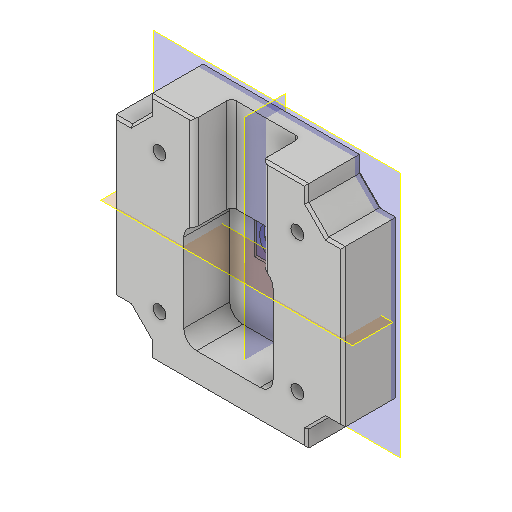
# Autodesk Inventor part: 20_Cube_Insert_SEEED_Xiao_Sense_Camera
Saved by Autodesk Inventor 2022 (Build 260153000, 153)
## iProperties
Created: 2019-07-01
Part Number: 20_Cube_Insert_SEEED_Xiao_Sense_Camera
Material: Generic
Document SubType Name: Modeling
Designer: diederichbenedict
Density: 1 g/cm^3
Appearance: Default
Author: diederichbenedict
Autodesk Inventor part; units mm, degrees
ref_plane "YZ Plane" through (0, 0, 0) normal (1, 0, 0) x (0, 1, 0)
ref_plane "Work Plane1" through (-56.3599, 0, 22) normal (0, 0, -1) x (-1, 0, 0)
sketch "Sketch1" plane through (-56.3599, 0, 22) normal (0, 0, -1) x (-1, 0, 0)
  line L0 (-4.0299, -0.3538) -> (-2.2322, 1.4439) construction
  arc A0 (-1.4439, 2.2322) -> (-2.2322, 1.4439) centre (-0.9299, 0.9299) ccw construction
  line L1 (-1.4439, 2.2322) -> (0.3538, 4.0299) construction
  line L2 (-37.8299, 42.8299) -> (-37.8299, 37.8299) construction
  line L3 (-37.8299, 37.8299) -> (-42.9208, 37.8299) construction
  line L4 (-37.8299, 42.2137) -> (-37.8299, 45.8299) construction
  line L5 (-37.8299, 45.8299) -> (-4.0299, 45.8299) construction
  line L6 (-4.0299, 45.8299) -> (-4.0299, 42.2137) construction
  line L7 (-4.0299, 4.0299) -> (0.3538, 4.0299) projected
  circle A1 centre (-20.9299, 20.9299) radius 17.5 projected
  line L8 (-20.9299, 58.9723) -> (17.1124, 20.9299) construction
  line L9 (17.1124, 20.9299) -> (-20.9299, -17.1124) construction
  line L10 (-20.9299, -17.1124) -> (-58.9723, 20.9299) construction
  line L11 (-58.9723, 20.9299) -> (-20.9299, 58.9723) construction
  line L12 (-20.9299, 58.9723) -> (-20.9299, -17.1124) construction
  line L13 (17.1124, 20.9299) -> (-58.9723, 20.9299) construction
  line L14 (-20.9299, 58.9723) -> (32.8701, 58.9723) construction
  line L15 (-43.4299, 43.4299) -> (1.5701, 43.4299) construction
  line L16 (1.5701, 43.4299) -> (1.5701, -1.5701) construction
  line L17 (1.5701, -1.5701) -> (-43.4299, -1.5701) construction
  line L18 (-43.4299, -1.5701) -> (-43.4299, 43.4299) construction
  line L19 (-43.4299, 43.4299) -> (1.5701, -1.5701) construction
  line L20 (1.5701, 43.4299) -> (-43.4299, -1.5701) construction
  line L21 (-43.4299, 5.3876) -> (-43.4299, 36.4723)
  line L22 (-43.4299, 36.4723) -> (-36.4723, 43.4299)
  line L23 (-36.4723, 43.4299) -> (-5.3876, 43.4299)
  line L24 (-5.3876, 43.4299) -> (1.5701, 36.4723)
  line L25 (1.5701, 36.4723) -> (1.5701, 5.3876)
  line L26 (1.5701, 5.3876) -> (-5.3876, -1.5701)
  line L27 (-5.3876, -1.5701) -> (-36.4723, -1.5701)
  line L28 (-36.4723, -1.5701) -> (-43.4299, 5.3876)
  line L29 (-4.0299, 42.2137) -> (-37.8299, 42.2137) projected
  line L30 (-4.0299, -0.3538) -> (-4.0299, 4.0299) projected
  circle A2 centre (-20.9299, 20.9299) radius 1.5
  line L31 (-10.9299, 10.9299) -> (-30.9299, 10.9299) construction
  line L32 (-30.9299, 10.9299) -> (-30.9299, 30.9299) construction
  line L33 (-30.9299, 30.9299) -> (-10.9299, 30.9299) construction
  line L34 (-10.9299, 30.9299) -> (-10.9299, 10.9299) construction
  line L35 (-10.9299, 10.9299) -> (-30.9299, 30.9299) construction
  line L36 (-30.9299, 10.9299) -> (-10.9299, 30.9299) construction
  circle A3 centre (-30.9299, 30.9299) radius 1.4
  circle A4 centre (-30.9299, 10.9299) radius 1.4
  circle A5 centre (-10.9299, 10.9299) radius 1.4
  line L37 (-45.8299, 37.8299) -> (-42.0723, 37.8299) construction
  line L38 (-42.1723, 37.7299) -> (-45.8299, 37.7299)
  line L39 (-45.8299, 37.7299) -> (-45.8299, 4.1299)
  line L40 (-45.8299, 4.1299) -> (-42.1723, 4.1299)
  line L41 (-42.1723, 4.1299) -> (-42.1723, 37.7299)
  line L42 (-45.8299, 4.0299) -> (-42.0723, 4.0299) construction
  line L43 (-45.8299, 37.8299) -> (-42.0723, 37.8299) projected
  line L44 (-37.7299, 45.8299) -> (-4.1299, 45.8299)
  line L45 (-4.1299, 45.8299) -> (-4.1299, 42.1723)
  line L46 (-4.1299, 42.1723) -> (-37.7299, 42.1723)
  line L47 (-37.7299, 42.1723) -> (-37.7299, 45.8299)
  line L48 (0.4701, 37.8299) -> (0.4701, 4.0299) construction
  line L49 (0.4701, 4.0299) -> (3.9701, 4.0299) construction
  line L50 (3.9701, 37.8299) -> (3.9701, 4.0299) construction
  line L51 (0.4701, 37.8299) -> (3.9701, 37.8299) construction
  line L52 (-45.8299, -3.9701) -> (-4.0299, -3.9701) construction
  line L53 (0.3124, 37.7299) -> (3.9701, 37.7299)
  line L54 (3.9701, 37.7299) -> (3.9701, 4.1299)
  line L55 (3.9701, 4.1299) -> (0.3124, 4.1299)
  line L56 (0.3124, 4.1299) -> (0.3124, 37.7299)
  line L57 (-4.1713, -0.3538) -> (-37.7299, -0.3538)
  line L58 (-37.7299, -0.3538) -> (-37.7299, -3.9701)
  line L59 (-37.7299, -3.9701) -> (-4.1713, -3.9701)
  line L60 (-4.1713, -3.9701) -> (-4.1713, -0.3538)
  point P0 (-37.8299, 4.0299)
  dimension "d18" = 53.8
  dimension "d19" = 45
  dimension "d20" = 53.8
  dimension "d21" = 45
  dimension "d22" = 45
  dimension "d30" = 20
  dimension "d31" = 20
  dimension "d32" = 2.8
  dimension "d33" = 2.8
  dimension "d34" = 2.8
  dimension "d35" = 3
  dimension "d36" = 0.1
  dimension "d37" = 0.1
  dimension "d38" = 0.1
  dimension "d39" = 0.1
  constraints: 86 end point, 21 point on line, 14 parallel, 8 perpendicular, 7 horizontal, 7 midpoint, 4 centre point, 4 coincident, 1 equal length
  measures "d18" distance of L8.start L8.end
  measures "d19" angle of L8 L14
  measures "d20" distance of L8.end L9.end
  measures "d21" distance of L16.end L17.end
  measures "d22" distance of L15.end L16.end
  measures "d30" distance of L32.end L33.end
  measures "d31" distance of L31.end L32.end
  measures "d32" diameter of A3
  measures "d33" diameter of A4
  measures "d34" diameter of A5
  measures "d35" diameter of A2
  measures "d36" distance between parallel lines of L38 L43
  measures "d37" distance between parallel lines of L40 L42
  measures "d38" distance between parallel lines of L45 L6
  measures "d39" distance between parallel lines of L4 L47
extrude "Extrusion1" add sketch "Sketch1" along normal blind 12 contours L30 L26 L57 L28 L41 L22 L46 L24 L56 L7 | L7 L26 L30 | L56 L24 L25 L26 | L26 L25 L24 L53 L54 L55 | L60 L59 L58 L57 L28 L27 L26 | L26 L27 L28 L57 | L46 L22 L29 L24 | L24 L29 L45 | L40 L39 L38 L22 L21 L28 | L28 L21 L22 L41 | L29 L22 L23 L24 | L24 L23 L22 L29 L47 L44 L45 | L47 L29 L22 | A1 | A2 | A3 | A4 | A5
sketch "Skizze4" plane through (-56.3599, 0, 10) normal (0, 0, -1) x (-1, 0, 0)
  line L0 (-37.7299, 42.1723) -> (-42.1723, 37.7299) projected
  line L1 (-42.1723, 37.7299) -> (-45.8299, 37.7299) projected
  line L2 (-45.8299, 37.7299) -> (-45.8299, 4.1299) construction
  line L3 (-45.8299, 4.1299) -> (-42.1723, 4.1299) projected
  line L4 (-42.1723, 4.1299) -> (-37.6885, -0.3538) projected
  line L5 (-37.6885, -0.3538) -> (-37.7299, -0.3538) projected
  line L6 (-37.7299, -0.3538) -> (-37.7299, -3.9701) projected
  line L7 (-37.7299, -3.9701) -> (-4.1713, -3.9701) construction
  line L8 (-4.1713, -3.9701) -> (-4.1713, -0.3538) projected
  line L9 (-4.1713, -0.3538) -> (0.3124, 4.1299) projected
  line L10 (0.3124, 4.1299) -> (3.9701, 4.1299) projected
  line L11 (3.9701, 4.1299) -> (3.9701, 37.7299) construction
  line L12 (3.9701, 37.7299) -> (0.3124, 37.7299) projected
  line L13 (0.3124, 37.7299) -> (-4.1299, 42.1723) projected
  line L14 (-4.1299, 42.1723) -> (-4.1299, 45.8299) projected
  line L15 (-4.1299, 45.8299) -> (-37.7299, 45.8299) construction
  line L16 (-37.7299, 45.8299) -> (-37.7299, 42.1723) projected
  line L17 (-37.9299, 46.0299) -> (-3.9299, 46.0299) construction
  line L18 (-3.9299, 46.0299) -> (-3.9299, 42.2551)
  line L19 (-3.9299, 42.2551) -> (0.3953, 37.9299)
  line L20 (0.3953, 37.9299) -> (4.1701, 37.9299)
  line L21 (4.1701, 37.9299) -> (4.1701, 3.9299) construction
  line L22 (4.1701, 3.9299) -> (0.3953, 3.9299)
  line L23 (0.3953, 3.9299) -> (-3.9713, -0.4367)
  line L24 (-3.9713, -0.4367) -> (-3.9713, -4.1701)
  line L25 (-3.9713, -4.1701) -> (-37.9299, -4.1701) construction
  line L26 (-37.9299, -4.1701) -> (-37.9299, -0.3953)
  line L27 (-37.9299, -0.3953) -> (-42.2551, 3.9299)
  line L28 (-42.2551, 3.9299) -> (-46.0299, 3.9299)
  line L29 (-46.0299, 3.9299) -> (-46.0299, 37.9299) construction
  line L30 (-46.0299, 37.9299) -> (-42.2551, 37.9299)
  line L31 (-42.2551, 37.9299) -> (-37.9299, 42.2551)
  line L32 (-37.9299, 42.2551) -> (-37.9299, 46.0299)
  line L33 (-45.8299, 37.7299) -> (-45.8299, 37.9299)
  line L34 (-4.1299, 45.8299) -> (-37.7299, 45.8299) projected
  line L35 (-37.7299, 45.8299) -> (-37.9299, 45.8299)
  line L36 (-4.1299, 45.8299) -> (-3.9299, 45.8299)
  line L37 (3.9701, 37.7299) -> (3.9701, 37.9299)
  line L38 (3.9701, 4.1299) -> (3.9701, 37.7299) projected
  line L39 (3.9701, 4.1299) -> (3.9701, 3.9299)
  line L40 (-4.1713, -3.9701) -> (-3.9713, -3.9701)
  line L41 (-37.7299, -3.9701) -> (-37.9299, -3.9701)
  line L42 (-45.8299, 4.1299) -> (-45.8299, 3.9299)
  point P0 (-56.3599, 0)
  dimension "d40" = 0.2
  constraints: 48 end point, 12 point on line, 4 perpendicular, 15 other
  measures "d40" distance between parallel lines of L15 L17
extrude "IM_offset" add sketch "Skizze4" against normal up to surface (12 mm away)
ref_plane "Arbeitsebene5" through (-35.4299, 3.9299, 22) normal (-1, 0, 0) x (0, 0, 1)
ref_plane "Arbeitsebene6" through (-18.4299, 20.9299, 22) normal (0, 1, 0) x (-1, 0, 0)
sketch "Skizze31" plane through (-56.3599, 0, 10) normal (0, 0, -1) x (-1, 0, 0)
  line L0 (3.9701, 3.9299) -> (3.9701, 37.9299) projected
  line L1 (3.9701, 37.9299) -> (0.3953, 37.9299) projected
  line L2 (0.3953, 37.9299) -> (-3.9299, 42.2551) projected
  line L3 (-3.9299, 42.2551) -> (-3.9299, 45.8299) projected
  line L4 (-3.9299, 45.8299) -> (-37.9299, 45.8299) projected
  line L5 (-37.9299, 45.8299) -> (-37.9299, 42.2551) projected
  line L6 (-37.9299, 42.2551) -> (-42.2551, 37.9299) projected
  line L7 (-42.2551, 37.9299) -> (-45.8299, 37.9299) projected
  line L8 (-45.8299, 37.9299) -> (-45.8299, 3.9299) projected
  line L9 (-42.2551, 3.9299) -> (-45.8299, 3.9299) projected
  line L10 (-37.9299, -0.3953) -> (-42.2551, 3.9299) projected
  line L11 (-37.9299, -3.9701) -> (-37.9299, -0.3953) projected
  line L12 (-3.9713, -3.9701) -> (-37.9299, -3.9701) projected
  line L13 (-3.9713, -3.9701) -> (-3.9713, -0.4367) projected
  line L14 (-3.9713, -0.4367) -> (0.3953, 3.9299) projected
  line L15 (0.3953, 3.9299) -> (3.9701, 3.9299) projected
  circle A0 centre (-20.9506, 20.9092) radius 3.75
  point P0 (-56.3599, 0)
  dimension "d181" = 7.5
  constraints: 1 centre point
  measures "d181" diameter of A0
extrude "Extrusion26" cut sketch "Skizze31" against normal blind 10 contours A0
chamfer "Fase2" distance 0.5 angle 45 33 edges at (-35.4299, 45.8299, 22) (-18.4299, 44.0425, 22) (-16.2673, 40.0925, 22) (-12.3173, 37.9299, 22) (-10.5299, 20.9299, 22) (-12.3173, 3.9299, 22) (-16.2673, 1.7673, 22) (-18.4299, -2.1827, 22) (-35.4092, -3.9701, 22) (-52.3885, -2.2034, 22) (-54.5718, 1.7466, 22) (-58.5425, 3.9299, 22) (-60.3299, 20.9299, 22) (-58.5425, 37.9299, 22) (-54.5925, 40.0925, 22) (-54.5718, 1.7466, 10) (-58.5425, 3.9299, 10) (-60.3299, 20.9299, 10) (-52.3885, -2.2034, 10) (-35.4092, -3.9701, 10) (-18.4299, -2.1827, 10) (-16.2673, 1.7673, 10) (-12.3173, 3.9299, 10) (-10.5299, 20.9299, 10) (-12.3173, 37.9299, 10) (-16.2673, 40.0925, 10) (-18.4299, 44.0425, 10) (-35.4299, 45.8299, 10) (-52.4299, 44.0425, 10) (-54.5925, 40.0925, 10) (-58.5425, 37.9299, 10) (-31.6592, 20.9092, 10) (-52.4299, 44.0425, 22)
ref_plane "Arbeitsebene9" through (-56.3599, 0, 11.5) normal (0, 0, -1) x (-1, 0, 0)
sketch "Skizze34" plane through (-56.3599, 0, 11.5) normal (0, 0, -1) x (-1, 0, 0)
  circle A0 centre (-20.9299, 20.9299) radius 4 projected
  line L0 (-16.6299, 25.2299) -> (-25.2299, 25.2299)
  line L1 (-25.2299, 25.2299) -> (-25.2299, 16.6299)
  line L2 (-25.2299, 16.6299) -> (-16.6299, 16.6299)
  line L3 (-16.6299, 16.6299) -> (-16.6299, 25.2299)
  line L4 (-16.6299, 25.2299) -> (-25.2299, 16.6299) construction
  line L5 (-25.2299, 25.2299) -> (-16.6299, 16.6299) construction
  point P0 (-56.3599, 0)
  dimension "d194" = 8.6
  dimension "d195" = 8.6
  constraints: 12 end point, 2 midpoint, 2 parallel, 1 horizontal, 1 perpendicular
  measures "d194" distance of L2.end L1.end
  measures "d195" distance of L1.end L0.end
extrude "Extrusion29" cut sketch "Skizze34" against normal through all contours A0 | L3 L2 L1 L0
sketch "Skizze35" plane through (-56.3599, 0, 22) normal (0, 0, 1) x (1, 0, 0)
  arc A0 (29.8299, 22.6299) -> (27.8299, 24.6299) centre (27.8299, 22.6299) ccw projected
  line L0 (27.8299, 24.6299) -> (14.0299, 24.6299) projected
  arc A1 (14.0299, 24.6299) -> (12.0299, 22.6299) centre (14.0299, 22.6299) ccw projected
  line L1 (12.0299, 22.6299) -> (12.0299, 22.5499) projected
  line L2 (12.0299, 22.5499) -> (13.3099, 22.5499) projected
  arc A2 (13.3099, 20.7499) -> (13.3099, 22.5499) centre (13.3099, 21.6499) ccw projected
  line L3 (13.3099, 20.7499) -> (12.0299, 20.7499) projected
  line L4 (12.0299, 20.7499) -> (12.0299, 20.0099) projected
  line L5 (12.0299, 20.0099) -> (13.3099, 20.0099) projected
  arc A3 (13.3099, 18.2099) -> (13.3099, 20.0099) centre (13.3099, 19.1099) ccw projected
  line L6 (13.3099, 18.2099) -> (12.0299, 18.2099) projected
  line L7 (12.0299, 18.2099) -> (12.0299, 17.4699) projected
  line L8 (12.0299, 17.4699) -> (13.3099, 17.4699) projected
  arc A4 (13.3099, 15.6699) -> (13.3099, 17.4699) centre (13.3099, 16.5699) ccw projected
  line L9 (13.3099, 15.6699) -> (12.0299, 15.6699) projected
  line L10 (12.0299, 15.6699) -> (12.0299, 14.9299) projected
  line L11 (12.0299, 14.9299) -> (13.3099, 14.9299) projected
  arc A5 (13.3099, 13.1299) -> (13.3099, 14.9299) centre (13.3099, 14.0299) ccw projected
  line L12 (13.3099, 13.1299) -> (12.0299, 13.1299) projected
  line L13 (12.0299, 13.1299) -> (12.0299, 12.3899) projected
  line L14 (12.0299, 12.3899) -> (13.3099, 12.3899) projected
  arc A6 (13.3099, 10.5899) -> (13.3099, 12.3899) centre (13.3099, 11.4899) ccw projected
  line L15 (13.3099, 10.5899) -> (12.0299, 10.5899) projected
  line L16 (12.0299, 10.5899) -> (12.0299, 9.8499) projected
  line L17 (12.0299, 9.8499) -> (13.3099, 9.8499) projected
  arc A7 (13.3099, 8.0499) -> (13.3099, 9.8499) centre (13.3099, 8.9499) ccw projected
  line L18 (13.3099, 8.0499) -> (12.0299, 8.0499) projected
  line L19 (12.0299, 8.0499) -> (12.0299, 7.3099) projected
  line L20 (12.0299, 7.3099) -> (13.3099, 7.3099) projected
  arc A8 (13.3099, 5.5099) -> (13.3099, 7.3099) centre (13.3099, 6.4099) ccw projected
  line L21 (13.3099, 5.5099) -> (12.0299, 5.5099) projected
  line L22 (12.0299, 5.5099) -> (12.0299, 5.4299) projected
  arc A9 (12.0299, 5.4299) -> (14.0299, 3.4299) centre (14.0299, 5.4299) ccw projected
  line L23 (14.0299, 3.4299) -> (27.8299, 3.4299) projected
  arc A10 (27.8299, 3.4299) -> (29.8299, 5.4299) centre (27.8299, 5.4299) ccw projected
  line L24 (29.8299, 5.4299) -> (29.8299, 5.5099) projected
  line L25 (29.8299, 5.5099) -> (28.5499, 5.5099) projected
  arc A11 (28.5499, 7.3099) -> (28.5499, 5.5099) centre (28.5499, 6.4099) ccw projected
  line L26 (28.5499, 7.3099) -> (29.8299, 7.3099) projected
  line L27 (29.8299, 7.3099) -> (29.8299, 8.0499) projected
  line L28 (29.8299, 8.0499) -> (28.5499, 8.0499) projected
  arc A12 (28.5499, 9.8499) -> (28.5499, 8.0499) centre (28.5499, 8.9499) ccw projected
  line L29 (28.5499, 9.8499) -> (29.8299, 9.8499) projected
  line L30 (29.8299, 9.8499) -> (29.8299, 10.5899) projected
  line L31 (29.8299, 10.5899) -> (28.5499, 10.5899) projected
  arc A13 (28.5499, 12.3899) -> (28.5499, 10.5899) centre (28.5499, 11.4899) ccw projected
  line L32 (28.5499, 12.3899) -> (29.8299, 12.3899) projected
  line L33 (29.8299, 12.3899) -> (29.8299, 13.1299) projected
  line L34 (29.8299, 13.1299) -> (28.5499, 13.1299) projected
  arc A14 (28.5499, 14.9299) -> (28.5499, 13.1299) centre (28.5499, 14.0299) ccw projected
  line L35 (28.5499, 14.9299) -> (29.8299, 14.9299) projected
  line L36 (29.8299, 14.9299) -> (29.8299, 15.6699) projected
  line L37 (29.8299, 15.6699) -> (28.5499, 15.6699) projected
  arc A15 (28.5499, 17.4699) -> (28.5499, 15.6699) centre (28.5499, 16.5699) ccw projected
  line L38 (28.5499, 17.4699) -> (29.8299, 17.4699) projected
  line L39 (29.8299, 17.4699) -> (29.8299, 18.2099) projected
  line L40 (29.8299, 18.2099) -> (28.5499, 18.2099) projected
  arc A16 (28.5499, 20.0099) -> (28.5499, 18.2099) centre (28.5499, 19.1099) ccw projected
  line L41 (28.5499, 20.0099) -> (29.8299, 20.0099) projected
  line L42 (29.8299, 20.0099) -> (29.8299, 20.7499) projected
  line L43 (29.8299, 20.7499) -> (28.5499, 20.7499) projected
  arc A17 (28.5499, 22.5499) -> (28.5499, 20.7499) centre (28.5499, 21.6499) ccw projected
  line L44 (28.5499, 22.5499) -> (29.8299, 22.5499) projected
  line L45 (29.8299, 22.5499) -> (29.8299, 22.6299) projected
  line L46 (29.8299, 22.5499) -> (12.0299, 22.5499)
  line L47 (12.0299, 22.5499) -> (12.0299, 5.4299)
  line L48 (12.0299, 5.4299) -> (29.8299, 5.4299)
  line L49 (29.8299, 5.4299) -> (29.8299, 22.5499)
  line L50 (27.8299, 2.6225) -> (14.0299, 2.6225)
  arc A18 (11.2225, 5.4299) -> (14.0299, 2.6225) centre (14.0299, 5.4299) ccw
  line L51 (11.2225, 5.4299) -> (11.2225, 6.3173)
  line L52 (11.2225, 6.3173) -> (13.3099, 6.3173)
  arc A19 (13.3099, 6.3173) -> (13.3099, 6.5025) centre (13.3099, 6.4099) ccw
  line L53 (13.3099, 6.5025) -> (11.2225, 6.5025)
  line L54 (11.2225, 6.5025) -> (11.2225, 8.8573)
  line L55 (11.2225, 8.8573) -> (13.3099, 8.8573)
  arc A20 (13.3099, 8.8573) -> (13.3099, 9.0425) centre (13.3099, 8.9499) ccw
  line L56 (13.3099, 9.0425) -> (11.2225, 9.0425)
  line L57 (11.2225, 9.0425) -> (11.2225, 11.3973)
  line L58 (11.2225, 11.3973) -> (13.3099, 11.3973)
  arc A21 (13.3099, 11.3973) -> (13.3099, 11.5825) centre (13.3099, 11.4899) ccw
  line L59 (13.3099, 11.5825) -> (11.2225, 11.5825)
  line L60 (11.2225, 11.5825) -> (11.2225, 13.9373)
  line L61 (11.2225, 13.9373) -> (13.3099, 13.9373)
  arc A22 (13.3099, 13.9373) -> (13.3099, 14.1225) centre (13.3099, 14.0299) ccw
  line L62 (13.3099, 14.1225) -> (11.2225, 14.1225)
  line L63 (11.2225, 14.1225) -> (11.2225, 16.4773)
  line L64 (11.2225, 16.4773) -> (13.3099, 16.4773)
  arc A23 (13.3099, 16.4773) -> (13.3099, 16.6625) centre (13.3099, 16.5699) ccw
  line L65 (13.3099, 16.6625) -> (11.2225, 16.6625)
  line L66 (11.2225, 16.6625) -> (11.2225, 19.0173)
  line L67 (11.2225, 19.0173) -> (13.3099, 19.0173)
  arc A24 (13.3099, 19.0173) -> (13.3099, 19.2025) centre (13.3099, 19.1099) ccw
  line L68 (13.3099, 19.2025) -> (11.2225, 19.2025)
  line L69 (11.2225, 19.2025) -> (11.2225, 21.5573)
  line L70 (11.2225, 21.5573) -> (13.3099, 21.5573)
  arc A25 (13.3099, 21.5573) -> (13.3099, 21.7425) centre (13.3099, 21.6499) ccw
  line L71 (13.3099, 21.7425) -> (11.2225, 21.7425)
  line L72 (11.2225, 21.7425) -> (11.2225, 22.6299)
  arc A26 (14.0299, 25.4373) -> (11.2225, 22.6299) centre (14.0299, 22.6299) ccw
  line L73 (14.0299, 25.4373) -> (27.8299, 25.4373)
  arc A27 (30.6373, 22.6299) -> (27.8299, 25.4373) centre (27.8299, 22.6299) ccw
  line L74 (30.6373, 22.6299) -> (30.6373, 21.7425)
  line L75 (30.6373, 21.7425) -> (28.5499, 21.7425)
  arc A28 (28.5499, 21.7425) -> (28.5499, 21.5573) centre (28.5499, 21.6499) ccw
  line L76 (28.5499, 21.5573) -> (30.6373, 21.5573)
  line L77 (30.6373, 21.5573) -> (30.6373, 19.2025)
  line L78 (30.6373, 19.2025) -> (28.5499, 19.2025)
  arc A29 (28.5499, 19.2025) -> (28.5499, 19.0173) centre (28.5499, 19.1099) ccw
  line L79 (28.5499, 19.0173) -> (30.6373, 19.0173)
  line L80 (30.6373, 19.0173) -> (30.6373, 16.6625)
  line L81 (30.6373, 16.6625) -> (28.5499, 16.6625)
  arc A30 (28.5499, 16.6625) -> (28.5499, 16.4773) centre (28.5499, 16.5699) ccw
  line L82 (28.5499, 16.4773) -> (30.6373, 16.4773)
  line L83 (30.6373, 16.4773) -> (30.6373, 14.1225)
  line L84 (30.6373, 14.1225) -> (28.5499, 14.1225)
  arc A31 (28.5499, 14.1225) -> (28.5499, 13.9373) centre (28.5499, 14.0299) ccw
  line L85 (28.5499, 13.9373) -> (30.6373, 13.9373)
  line L86 (30.6373, 13.9373) -> (30.6373, 11.5825)
  line L87 (30.6373, 11.5825) -> (28.5499, 11.5825)
  arc A32 (28.5499, 11.5825) -> (28.5499, 11.3973) centre (28.5499, 11.4899) ccw
  line L88 (28.5499, 11.3973) -> (30.6373, 11.3973)
  line L89 (30.6373, 11.3973) -> (30.6373, 9.0425)
  line L90 (30.6373, 9.0425) -> (28.5499, 9.0425)
  arc A33 (28.5499, 9.0425) -> (28.5499, 8.8573) centre (28.5499, 8.9499) ccw
  line L91 (28.5499, 8.8573) -> (30.6373, 8.8573)
  line L92 (30.6373, 8.8573) -> (30.6373, 6.5025)
  line L93 (30.6373, 6.5025) -> (28.5499, 6.5025)
  arc A34 (28.5499, 6.5025) -> (28.5499, 6.3173) centre (28.5499, 6.4099) ccw
  line L94 (28.5499, 6.3173) -> (30.6373, 6.3173)
  line L95 (30.6373, 6.3173) -> (30.6373, 5.4299)
  arc A35 (27.8299, 2.6225) -> (30.6373, 5.4299) centre (27.8299, 5.4299) ccw
  line L96 (30.6373, 6.3173) -> (11.2225, 6.3173)
  line L97 (11.2225, 6.3173) -> (11.2225, 21.7425)
  line L98 (11.2225, 21.7425) -> (30.6373, 21.7425)
  line L99 (30.6373, 21.7425) -> (30.6373, 6.3173)
  point P0 (56.3599, 0)
  point P1 (11.2225, 21.5573)
  point P2 (11.2225, 19.2025)
  point P3 (11.2225, 19.0173)
  point P4 (11.2225, 16.6625)
  point P5 (11.2225, 16.4773)
  point P6 (11.2225, 14.1225)
  point P7 (11.2225, 13.9373)
  point P8 (11.2225, 11.5825)
  point P9 (11.2225, 11.3973)
  point P10 (11.2225, 9.0425)
  point P11 (11.2225, 8.8573)
  point P12 (11.2225, 6.5025)
  point P13 (11.2225, 6.3173)
  point P14 (30.6373, 6.5025)
  point P15 (30.6373, 19.2025)
  constraints: 108 end point, 36 point on circle, 18 centre point, 4 parallel, 2 horizontal, 2 perpendicular, 63 other
extrude "Extrusion30" cut sketch "Skizze35" against normal blind 10
sketch "Skizze36" plane through (-52.4299, 45.8299, 10.5) normal (0, 1, 0) x (1, 0, 0)
  arc A0 (20.5, -9.5) -> (21.5, -8.5) centre (20.5, -8.5) ccw projected
  arc A1 (12.5, -8.5) -> (13.5, -9.5) centre (13.5, -8.5) ccw projected
  arc A2 (21.5, -7.33) -> (20.5, -6.33) centre (20.5, -7.33) ccw projected
  arc A3 (13.5, -6.33) -> (12.5, -7.33) centre (13.5, -7.33) ccw projected
  line L0 (20.5, -8.5) -> (13.5, -8.5)
  line L1 (13.5, -8.5) -> (13.5, -7.33)
  line L2 (13.5, -7.33) -> (20.5, -7.33)
  line L3 (20.5, -7.33) -> (20.5, -8.5)
  line L4 (9.5, -12.5) -> (24.5, -12.5)
  line L5 (24.5, -12.5) -> (24.5, -3.33)
  line L6 (24.5, -3.33) -> (9.5, -3.33)
  line L7 (9.5, -3.33) -> (9.5, -12.5)
  point P0 (52.4299, 10.5)
  dimension "d200" = 4
  constraints: 16 end point, 4 parallel, 2 perpendicular, 1 horizontal, 3 other
  measures "d200" distance between parallel lines of L0 L4
ref_plane "Arbeitsebene10" through (-41.4299, 4.7299, 19.7) normal (0, -1, 0) x (1, 0, 0)
extrude "Extrusion31" cut sketch "Skizze36" against normal up to surface (41.1 mm away) contours L0 L1 L2 L3 | L7 L6 L5 L4
fillet "Rundung3" radius 1 4 edges at (-27.9299, 35.3512, 22) (-27.9299, 35.6012, 13.83) (-42.9299, 35.3512, 22) (-42.9299, 35.6012, 13.83)
sketch "Skizze37" plane through (-56.3599, 0, 22) normal (0, 0, 1) x (1, 0, 0)
  line L0 (12.4299, 45.3299) -> (12.4299, 24.9368) projected
  line L1 (4.4299, 45.3299) -> (12.4299, 45.3299) projected
  line L2 (4.4299, 42.048) -> (4.4299, 45.3299) projected
  line L3 (-0.1882, 37.4299) -> (4.4299, 42.048) projected
  line L4 (-3.4701, 37.4299) -> (-0.1882, 37.4299) projected
  line L5 (-3.4701, 4.4299) -> (-3.4701, 37.4299) projected
  line L6 (-0.1882, 4.4299) -> (-3.4701, 4.4299) projected
  line L7 (4.4713, -0.2296) -> (-0.1882, 4.4299) projected
  line L8 (4.4713, -3.4701) -> (4.4713, -0.2296) projected
  line L9 (37.4299, -3.4701) -> (4.4713, -3.4701) projected
  line L10 (37.4299, -0.1882) -> (37.4299, -3.4701) projected
  line L11 (42.048, 4.4299) -> (37.4299, -0.1882) projected
  line L12 (45.3299, 4.4299) -> (42.048, 4.4299) projected
  line L13 (45.3299, 37.4299) -> (45.3299, 4.4299) projected
  line L14 (42.048, 37.4299) -> (45.3299, 37.4299) projected
  line L15 (37.4299, 42.048) -> (42.048, 37.4299) projected
  line L16 (37.4299, 45.3299) -> (37.4299, 42.048) projected
  line L17 (29.4299, 45.3299) -> (37.4299, 45.3299) projected
  line L18 (29.4299, 24.9368) -> (29.4299, 45.3299) projected
  arc A0 (30.6373, 22.6299) -> (29.4299, 24.9368) centre (27.8299, 22.6299) ccw projected
  line L19 (30.6373, 22.6299) -> (30.6373, 5.4299) projected
  arc A1 (27.8299, 2.6225) -> (30.6373, 5.4299) centre (27.8299, 5.4299) ccw projected
  line L20 (27.8299, 2.6225) -> (14.0299, 2.6225) projected
  arc A2 (11.2225, 5.4299) -> (14.0299, 2.6225) centre (14.0299, 5.4299) ccw projected
  line L21 (11.2225, 5.4299) -> (11.2225, 22.6299) projected
  arc A3 (12.4299, 24.9368) -> (11.2225, 22.6299) centre (14.0299, 22.6299) ccw projected
  circle A4 centre (20.9299, 20.9299) radius 4 projected
  line L22 (35.9299, 35.9299) -> (5.9299, 35.9299) construction
  line L23 (5.9299, 35.9299) -> (5.9299, 5.9299) construction
  line L24 (5.9299, 5.9299) -> (35.9299, 5.9299) construction
  line L25 (35.9299, 5.9299) -> (35.9299, 35.9299) construction
  line L26 (35.9299, 35.9299) -> (5.9299, 5.9299) construction
  line L27 (5.9299, 35.9299) -> (35.9299, 5.9299) construction
  point P0 (56.3599, 0)
  dimension "d204" = 30
  dimension "d205" = 30
  constraints: 12 end point, 4 coincident, 2 midpoint, 2 parallel, 1 horizontal, 1 perpendicular
  measures "d204" distance of L24.end L23.end
  measures "d205" distance of L23.end L22.end
hole "Bohrung2" at (-20.4299, 5.9299, 22) at (-50.4299, 5.9299, 22) at (-50.4299, 35.9299, 22) at (-20.4299, 35.9299, 22) direction (0, 0, -1) diameter 2.8 end through all
body "Solid1"
